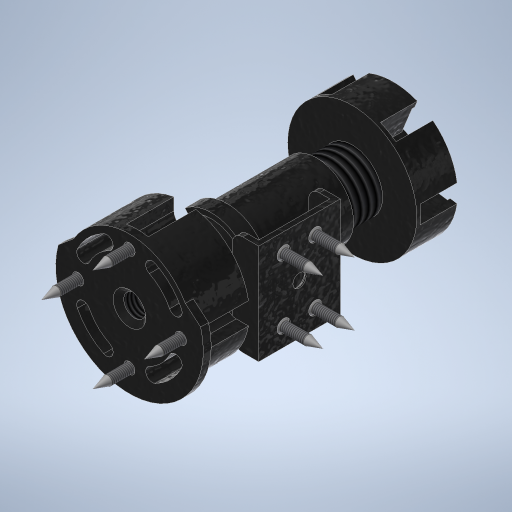
# Autodesk Inventor part: Adjustable leg  BT18 clip included
Saved by Autodesk Inventor 2024 (Build 280153000, 153)
## iProperties
Perskaiciuoti: 1
Category: Legs and supports
Created: 2006-11-23
Document SubType Name: Modeling
Designer: G.K.
Description: Adjustable leg
Authority: Design by UAB Čeli APS
Part Number: Adjustable leg  BT18 clip included
Mass: 31.9573 g
Surface Area: 217.096 cm^2
Volume: 31.9573 cm^3
Density: 1 g/cm^3
Material: Generic
Appearance: Fine Textured - Black
Pavadinimas: Koja
Šifras: Koja 001
Mase: 0.03195727
Author: G.K.
Title: Ajustable leg
Subject: Legs
Keywords: leg, adjustable, black
Comments: Ajustable leg, adjustable, black
Revision Number: 1
Autodesk Inventor part; units mm, degrees
ref_plane "YZ Plane" through (0, 0, 0) normal (1, 0, 0) x (0, 1, 0)
sketch "Sketch1" plane through (0, 0, 0) normal (1, 0, 0) x (0, 1, 0)
  line L0 (-14.2, 0) -> (85.2, 0) projected
  line L1 (0, 33.6) -> (0, -5.6) projected
  line L2 (71, 10.5) -> (71, 14)
  line L3 (71, 14) -> (21, 14)
  line L4 (21, 14) -> (21, 24.5)
  line L5 (21, 24.5) -> (3, 24.5)
  line L6 (3, 24.5) -> (3, 28)
  line L7 (3, 28) -> (0, 28)
  line L8 (0, 28) -> (0, 0)
  line L9 (71, 10.5) -> (53, 10.5)
  line L10 (53, 10.5) -> (53, 12)
  line L11 (53, 12) -> (3, 12)
  line L12 (3, 12) -> (3, 7)
  line L13 (3, 7) -> (9, 7)
  line L14 (9, 7) -> (9, 0)
  dimension "d139" = 24
  dimension "d0" = 71
  dimension "d1" = 68
  dimension "d2" = 18
  dimension "d3" = 56
  dimension "d4" = 49
  dimension "d5" = 3
  dimension "d6" = 21
  dimension "d7" = 28
  dimension "d8" = 21
  dimension "d9" = 24
  dimension "d11" = 62
  dimension "d12" = 14
  constraints: 26 end point, 6 parallel, 5 perpendicular, 4 point on line, 1 vertical
  measures "d0" distance between parallel lines of L2 L1
  measures "d1" distance between parallel lines of L12 L2
  measures "d2" distance of L2.start L9.end
  measures "d3" diameter of L7 L0
  measures "d4" diameter of L5 L0
  measures "d5" distance between parallel lines of L6 L8
  measures "d6" distance between parallel lines of L4 L8
  measures "d7" diameter of L3 L0
  measures "d8" diameter of L9 L0
  measures "d9" diameter of L11 L0
  measures "d11" distance between parallel lines of L14 L2
  measures "d12" diameter of L13 L0
revolve "Revolution1" add sketch "Sketch1" angle 360 about axis through (0, 0, 0) along (0, 1, 0)
sketch "Sketch2" plane through (0, 21, 0) normal (0, 1, 0) x (1, 0, 0)
  circle A0 centre (0, 0) radius 24.5 projected
  circle A1 centre (0, 0) radius 19.5 construction
  line L0 (0, 39.2) -> (0, -39.2) projected
  point P0 (0, 19.5)
  dimension "d14" = 39
  constraints: 1 coincident, 1 point on line, 1 vertical alignment, 2 other
hole "Hole1" at (0, 21, -19.5) direction (0, -1, 0) diameter 4.3 end through all
sketch "Sketch3" plane through (0, 21, 0) normal (0, 1, 0) x (1, 0, 0)
  circle A0 centre (0, 19.5) radius 2.15 projected
  circle A1 centre (0, 0) radius 24.5 projected
  arc A2 (-4.15, 19.5) -> (4.15, 19.5) centre (0, 19.5) ccw
  line L0 (-4.15, 19.5) -> (-4.15, 24.146)
  line L1 (4.15, 19.5) -> (4.15, 24.146)
  dimension "d22" = 8.3
  constraints: 4 end point, 4 point on circle, 2 tangent, 1 centre point, 1 coincident, 1 parallel, 1 vertical
  measures "d22" distance between parallel lines of L1 L0
extrude "Extrusion1" cut sketch "Sketch3" against normal blind 18 contours L1 A2 L0 A1 picked at (-3.4012, 21.3817)
hole "Hole2" at (0, 0, 0) direction (0, 1, 0) diameter 8.376 depth 20 tip angle 118 thread size "M10x1.5" class "6H" standard "ISO Metric profile"
thread "Thread1" size "M22x3" class "6H" standard "ISO Metric profile" full length
sketch "Sketch4" plane through (0, 0, 0) normal (0, -1, 0) x (1, 0, 0)
  circle A0 centre (0, 0) radius 28 projected
  arc A1 (7.1625, -20.8014) -> (20.8014, -7.1625) centre (0, 0) ccw
  arc A2 (5.5347, -16.0738) -> (16.0738, -5.5347) centre (0, 0) ccw
  arc A3 (4.15, -24.146) -> (24.146, -4.15) centre (0, 0) ccw projected
  line L0 (0, 39.2) -> (0, -39.2) projected
  line L1 (16.0738, -5.5347) -> (20.8014, -7.1625)
  line L2 (5.5347, -16.0738) -> (7.1625, -20.8014)
  line L3 (16.0738, -5.5347) -> (0, 0) construction
  line L4 (0, 0) -> (5.5347, -16.0738) construction
  dimension "d39" = 5
  dimension "d40" = 2.5
  dimension "d43" = 52
  dimension "d44" = 19
  constraints: 8 end point, 5 point on circle, 2 centre point, 2 coincident, 2 collinear, 1 point on line
  measures "d39" radial gap between concentric circles of A1 A2
  measures "d40" radial gap between concentric circles of A1 A3
  measures "d43" angle of L4 L3
  measures "d44" angle of L0 L4
extrude "Extrusion2" cut sketch "Sketch4" against normal blind 18 contours L2 A2 L1 A1
full round fillet "Fillet1" first side at (8.7138, 6, -20.2008) centre faces at (19.2255, 6, -6.6199) second side at (6.7334, 12, -15.6097)
full round fillet "Fillet2" first side at (8.4969, 6, -20.2929) centre faces at (6.0773, 6, -17.6497) second side at (14.7098, 6, -8.5219)
pattern_circular "Circular Pattern2" count 4 over 360 about axis through (0, 46, 0) along (0, -1, 0) of "Hole1", "Extrusion1", "Extrusion2", "Fillet1", "Fillet2"
chamfer "Chamfer1" distance 2 angle 45 1 edges at (0, 0, 4.188)
sketch "Sketch5" plane through (0, 3, 0) normal (0, 1, 0) x (1, 0, 0)
  arc A0 (24.146, 4.15) -> (4.15, 24.146) centre (0, 0) ccw projected
  line L0 (24.146, 4.15) -> (19.5, 4.15) projected
  arc A1 (-24.146, -4.15) -> (-4.15, -24.146) centre (0, 0) ccw projected
  line L1 (-24.146, -4.15) -> (-19.5, -4.15) projected
  line L2 (-19.5, 4.15) -> (-24.146, 4.15) projected
  circle A2 centre (0, 0) radius 28 projected
  line L3 (-27, -7.4162) -> (-21.1972, -12.2853)
  line L4 (0, 39.2) -> (0, -39.2) projected
  line L5 (27, -7.4162) -> (21.1972, -12.2853)
  arc A3 (-21.1972, -12.2853) -> (21.1972, -12.2853) centre (0, 0) ccw
  arc A4 (-27, -7.4162) -> (27, -7.4162) centre (0, 0) ccw
  dimension "d53" = 27
  dimension "d54" = 50
  constraints: 7 end point, 6 point on circle, 2 centre point, 2 coincident, 2 symmetric about line, 2 other
  measures "d53" distance from line of L4 L3.start
  measures "d54" angle of L3 L4
extrude "Extrusion3" cut sketch "Sketch5" against normal through all contours A1 A3 L4 A2 L3 | A3 L5 A2 L4 picked at (-24.3219, -10.92) picked at (24.3219, -10.92)
sketch "Sketch6" plane through (0, 0, 0) normal (0, 0, 1) x (1, 0, 0)
  line L0 (0, 22.894) -> (0, 122.294)
  line L1 (-28.3275, 84.5) -> (5.9725, 84.5)
  line L2 (-11.5, 29) -> (-11.5, 84.5)
  line L3 (-11.5, 84.5) -> (-24.5, 84.5)
  line L4 (-24.5, 84.5) -> (-24.5, 86)
  line L5 (-24.5, 86) -> (-11.5, 86)
  line L6 (-11.5, 86) -> (-11.5, 100)
  line L7 (-11.5, 100) -> (-9.25, 100)
  line L8 (-9.25, 100) -> (-9.25, 86)
  line L9 (-9.25, 86) -> (0, 86)
  line L10 (0, 84.5) -> (-9.5, 84.5)
  line L11 (-9.5, 84.5) -> (-9.5, 29)
  line L12 (-9.5, 29) -> (-11.5, 29)
  line L13 (0, 84.5) -> (0, 86)
  line L14 (14, 71) -> (-14, 71) projected
  point P0 (0, 0)
  dimension "d57" = 23
  dimension "d58" = 18.5
  dimension "d59" = 19
  dimension "d60" = 71
  dimension "d61" = 14
  dimension "d62" = 49
  dimension "d63" = 1.5
  dimension "d64" = 23
  dimension "d68" = 13.5
  constraints: 28 end point, 6 parallel, 5 collinear, 4 perpendicular, 3 point on line
  measures "d57" diameter of L2 L0
  measures "d58" diameter of L8 L0
  measures "d59" diameter of L11 L0
  measures "d60" distance between parallel lines of L12 L7
  measures "d61" distance between parallel lines of L7 L5
  measures "d62" diameter of L4 L0
  measures "d63" distance between parallel lines of L5 L1
  measures "d64" diameter of L6 L0
  measures "d68" distance between parallel lines of L3 L14
revolve "Revolution2" add sketch "Sketch6" angle 360 about axis through (0, 22.894, 0) along (0, 1, 0) separate body contours L1 L4 L5 L6 L7 L8 L9 L0 | L11 L14 L2 L1 | L11 L12 L2 L14
thread "Thread2" size "M24x3" class "6g" standard "ANSI Metric M Profile" full length
sketch "Sketch7" plane through (0, 86, 0) normal (0, 1, 0) x (1, 0, 0)
  circle A0 centre (0, 0) radius 11.5
  circle A1 centre (0, 0) radius 24.5
  arc A2 (7.2068, 21.8417) -> (-7.2068, 21.8417) centre (0, 0) ccw
  line L0 (-5.3569, 13.2587) -> (-9.1779, 22.716)
  line L1 (5.3369, 13.2093) -> (9.1779, 22.716)
  line L2 (-5.3569, 13.2587) -> (0, 0) construction
  line L3 (0, 0) -> (5.3369, 13.2093) construction
  line L4 (-5.3569, 13.2587) -> (-4.308, 10.6626)
  line L5 (5.3369, 13.2093) -> (4.308, 10.6626)
  line L6 (7.2068, 21.8417) -> (2.8804, 11.1334)
  line L7 (-7.2068, 21.8417) -> (-2.8804, 11.1334)
  dimension "d72" = 1.5
  dimension "d73" = 44
  dimension "d74" = 1.5
  dimension "d75" = 1.5
  constraints: 16 end point, 8 point on circle, 3 centre point, 2 collinear, 2 parallel, 2 point on line, 1 coincident
  measures "d72" radial gap between concentric circles of A2 A1
  measures "d73" angle of L3 L2
  measures "d74" distance between parallel lines of L5 L6
  measures "d75" distance between parallel lines of L7 L2
extrude "Extrusion4" add sketch "Sketch7" along normal up to surface (14 mm away) contours A0 L6 A2 L7 L4 L0 A1 L1 L5 bodies 2
pattern_circular "Circular Pattern3" count 6 over 360 about axis through (0, 85.25, 0) along (0, 1, 0) of "Extrusion4" bodies 2
sketch "Sketch8" plane through (0, 0, 0) normal (1, 0, 0) x (0, 1, 0)
  line L0 (99, 21.8417) -> (105.0942, 21.8417)
  line L1 (105.0942, 21.8417) -> (105.0942, 11.5)
  line L2 (105.0942, 11.5) -> (99, 11.5)
  line L3 (99, 11.5) -> (99, 21.8417)
  line L4 (86, 11.5) -> (100, 11.5) projected
  line L5 (100, 11.1334) -> (100, 21.8417) projected
  line L6 (86, 21.8417) -> (100, 21.8417) projected
  line L7 (-21.0188, 0) -> (126.113, 0) projected
  point P0 (0, 0)
  dimension "d81" = 1
  constraints: 8 end point, 2 collinear, 2 parallel, 1 horizontal, 1 perpendicular
  measures "d81" distance between parallel lines of L3 L5
revolve "Revolution3" cut sketch "Sketch8" angle 360 about axis through (0, -10, 0) along (0, 1, 0) bodies 2
revolve "Revolution4" [suppressed]
sketch "Sketch10" plane through (0, -24.4, 0) normal (0, -1, 0) x (1, 0, 0)
  circle A0 centre (0, 0) radius 8 projected
  line L0 (9.2376, -0.0209) -> (4.6007, -8.0104)
  line L1 (4.6007, -8.0104) -> (-4.6369, -7.9895)
  line L2 (-4.6369, -7.9895) -> (-9.2376, 0.0209)
  line L3 (-9.2376, 0.0209) -> (-4.6007, 8.0104)
  line L4 (-4.6007, 8.0104) -> (4.6369, 7.9895)
  line L5 (4.6369, 7.9895) -> (9.2376, -0.0209)
  constraints: 12 end point, 1 coincident, 1 tangent, 13 other
extrude "Extrusion5" [suppressed]
thread "Thread3" size "M10x1.5" class "6g" standard "ANSI Metric M Profile" full length
sketch "Sketch14" plane through (0, -18, 0) normal (0, 1, 0) x (1, 0, 0)
  circle A0 centre (0, 0) radius 5 projected
  circle A1 centre (0, 0) radius 7.25 projected
  circle A2 centre (0, 0) radius 5
  dimension "d102" = 10
  constraints: 1 centre point, 1 coincident
  measures "d102" diameter of A2
extrude "Extrusion6" [suppressed]
sketch "Sketch15" plane through (0, 0, 0) normal (1, 0, 0) x (0, 1, 0)
  line L0 (3, -23.7) -> (3, -18.8) construction
  line L1 (6.6298, -19.5) -> (-17.1702, -19.5)
  line L2 (3, -19.5) -> (3, -23)
  line L3 (3, -23) -> (2.5, -23)
  line L4 (2.5, -23) -> (0.75, -21.25)
  line L5 (0.75, -21.25) -> (-8.276, -21.25)
  line L6 (-8.276, -21.25) -> (-14, -19.5)
  line L7 (0, -21.65) -> (0, -17.35) projected
  line L8 (0, -19.5) -> (3.4682, -19.5) construction
  line L9 (3, -24.146) -> (3, -19.5) projected
  point P0 (0, 0)
  dimension "d105" = 3.5
  dimension "d106" = 7
  dimension "d107" = 0.5
  dimension "d108" = 45
  dimension "d109" = 17
  dimension "d110" = 17
  dimension "d111" = 9.026
  constraints: 16 end point, 3 collinear, 3 perpendicular, 2 point on line, 1 midpoint, 1 parallel
  measures "d105" diameter of L5 L1
  measures "d106" diameter of L3 L1
  measures "d107" distance from line of L3.end L2
  measures "d108" angle of L4 L2
  measures "d109" distance from line of L6.end L2
  measures "d110" angle of L6 L1
  measures "d111" distance of L4.end L5.end
revolve "Revolution8" add sketch "Sketch15" angle 360 about axis through (0, 6.6298, -19.5) along (0, -1, 0) separate body
sketch "Sketch16" plane through (0, 0, 0) normal (1, 0, 0) x (0, 1, 0)
  line L0 (0.84, -19.5) -> (3.36, -19.5)
  line L1 (1.2, -19.5) -> (1.2, -18.5104)
  line L2 (1.2, -18.5104) -> (3, -17)
  line L3 (3, -17) -> (3, -19.5)
  line L4 (3, -21.65) -> (3, -17.35) projected
  point P0 (0, 0)
  point P1 (3, -19.5)
  dimension "d113" = 40
  dimension "d114" = 1.8
  dimension "d115" = 2.5
  constraints: 8 end point, 2 perpendicular, 2 point on line, 1 midpoint
  measures "d113" angle of L2 L0
  measures "d114" distance between parallel lines of L1 L3
  measures "d115" distance from line of L0 L2.end
extrude "Extrusion7" cut sketch "Sketch16" along normal mid plane 1 bodies 3
pattern_circular "Circular Pattern4" count 4 over 360 about axis through (0, -3.763, -19.5) along (0, -1, 0) of "Extrusion7" bodies 3
thread "Thread4" size "M4x0.7" class "6g" standard "ANSI Metric M Profile" full length
ref_plane "Work Plane2" through (0, 31, 0) normal (0, -1, 0) x (1, 0, 0)
sketch "Sketch18" plane through (0, 31, 0) normal (0, -1, 0) x (1, 0, 0)
  arc A0 (-8.6603, -11) -> (-8.6603, 11) centre (0, 0) ccw
  arc A1 (-9.8974, -12.5714) -> (-9.8974, 12.5714) centre (0, 0) ccw
  line L0 (18, -10) -> (18, 10)
  line L1 (14, -6.4724) -> (14, 14.1834) construction
  line L2 (21, 10) -> (21, -10) construction
  line L3 (18, -7.5) -> (14.1333, -7.5)
  line L4 (14.1333, 7.5) -> (18, 7.5)
  line L5 (27.1795, 0) -> (0, 34.0769) construction
  line L6 (-8.6603, -11) -> (-9.8974, -12.5714)
  line L7 (-8.6603, 11) -> (-9.8974, 12.5714)
  point P0 (0, 0)
  point P1 (18, 0)
  point P2 (18, 0)
  point P3 (27.1795, 0)
  point P4 (0, 34.0769)
  dimension "d129" = 2
  dimension "d130" = 28
  dimension "d131" = 7
  dimension "d132" = 15
  dimension "d133" = 22
  constraints: 14 end point, 6 point on circle, 3 point on line, 2 centre point, 2 perpendicular, 1 coincident, 1 midpoint, 1 parallel, 1 tangent, 3 other
  measures "d129" radial gap between concentric circles of A1 A0
  measures "d130" diameter of A0
  measures "d131" distance between parallel lines of L1 L2
  measures "d132" distance between parallel lines of L4 L3
  measures "d133" distance of L7.start L6.start
extrude "Extrusion8" add sketch "Sketch18" against normal blind 6 separate body
sketch "Sketch19" plane through (0, 31, 0) normal (0, -1, 0) x (1, 0, 0)
  line L0 (18, -7.5) -> (18, 7.5) projected
  arc A0 (14.1333, 7.5) -> (-9.8974, 12.5714) centre (0, 0) ccw projected
  line L1 (21, 10) -> (18, 10)
  line L2 (18, 10) -> (18, -10)
  line L3 (18, -10) -> (21, -10)
  line L4 (21, -10) -> (21, 10)
  point P0 (21, 0)
  dimension "d136" = 20
  dimension "d137" = 3
  constraints: 8 end point, 2 parallel, 1 collinear, 1 horizontal, 1 horizontal alignment, 1 midpoint, 1 perpendicular
  measures "d136" distance of L3.end L1.start
  measures "d137" distance of L1.start L1.end
extrude "Extrusion9" add sketch "Sketch19" along normal blind 3 and the other way blind 24 bodies 4
sketch "Sketch20" plane through (0, 28, 0) normal (0, -1, 0) x (1, 0, 0)
  line L0 (18, 10) -> (18, -10) projected
  line L1 (23, 19) -> (17, 19)
  line L2 (13, 15) -> (13, -15)
  line L3 (17, -19) -> (23, -19)
  line L4 (23, -19) -> (23, 19)
  arc A0 (17, 19) -> (13, 15) centre (17, 15) ccw
  arc A1 (13, -15) -> (17, -19) centre (17, -15) ccw
  point P0 (0, 0)
  point P1 (13, -19)
  point P2 (13, 19)
  point P3 (23, 0)
  dimension "d142" = 10
  dimension "d143" = 38
  dimension "d144" = 5
  dimension "d145" = 4
  constraints: 8 end point, 4 point on circle, 4 point on line, 4 tangent, 2 centre point, 2 parallel, 1 equal radius, 1 horizontal, 1 horizontal alignment, 1 midpoint, 1 perpendicular
  measures "d142" distance of L3.end point (13, -19)
  measures "d143" distance of point (13, -19) point (13, 19)
  measures "d144" distance between parallel lines of L4 L0
  measures "d145" radius of A0
extrude "Extrusion10" add sketch "Sketch20" along normal blind 2 and the other way blind 29 separate body
sketch "Sketch21" plane through (23, 26, -19) normal (0, 0, -1) x (-1, 0, 0)
  line L0 (0, 31) -> (0, 0) projected
  line L1 (6, 0) -> (0, 0) projected
  line L2 (0, 31) -> (6, 31) projected
  line L3 (2, 29) -> (13.1026, 29)
  line L4 (13.1026, 29) -> (13.1026, 2)
  line L5 (13.1026, 2) -> (2, 2)
  line L6 (2, 2) -> (2, 29)
  point P0 (23, -26)
  dimension "d150" = 2
  dimension "d151" = 2
  dimension "d152" = 2
  constraints: 8 end point, 2 parallel, 1 horizontal, 1 perpendicular
  measures "d150" distance between parallel lines of L5 L1
  measures "d151" distance between parallel lines of L2 L3
  measures "d152" distance between parallel lines of L0 L6
extrude "Extrusion11" cut sketch "Sketch21" against normal through all bodies 5
sketch "Sketch22" plane through (21, 28, -19) normal (-1, 0, 0) x (0, 0, 1)
  line L0 (38, 27) -> (38, 0) projected
  line L1 (7, 19.5) -> (31, 19.5)
  line L2 (31, 19.5) -> (31, 7.5)
  line L3 (31, 7.5) -> (7, 7.5)
  line L4 (7, 7.5) -> (7, 19.5)
  line L5 (7, 19.5) -> (31, 7.5) construction
  line L6 (31, 19.5) -> (7, 7.5) construction
  line L7 (34, 0) -> (4, 0) projected
  point P0 (19, -28)
  point P1 (19, 13.5)
  point P2 (19, 13.5)
  point P3 (19, 0)
  point P4 (19, 13.5)
  point P5 (38, 13.5)
  dimension "d155" = 24
  dimension "d156" = 12
  constraints: 12 end point, 6 midpoint, 2 parallel, 1 horizontal, 1 horizontal alignment, 1 perpendicular, 1 vertical alignment
  measures "d155" distance of L2.end L3.end
  measures "d156" distance of L1.end L2.end
hole "Hole3" at (21, 35.5, -12) at (21, 41.5, 0) at (21, 47.5, -12) at (21, 47.5, 12) at (21, 35.5, 12) direction (1, 0, 0) diameter 5 end through all countersink diameter 8 countersink angle 90 bodies 5
ref_plane "Work Plane3" through (71.05, 47.5, -12) normal (0, 0, -1) x (-1, 0, 0)
sketch "Sketch23" plane through (71.05, 47.5, -12) normal (0, 0, -1) x (-1, 0, 0)
  line L0 (50.05, -4.2) -> (50.05, 0.7) construction
  line L1 (53.45, 0) -> (29.65, 0)
  line L2 (50.05, 0) -> (50.05, -3.5)
  line L3 (50.05, -3.5) -> (49.55, -3.5)
  line L4 (49.55, -3.5) -> (47.8, -1.75)
  line L5 (47.8, -1.75) -> (38.774, -1.75)
  line L6 (38.774, -1.75) -> (33.05, 0)
  line L7 (50.05, 4) -> (50.05, -4) projected
  point P0 (71.05, -47.5)
  point P1 (50.05, 0)
  dimension "d165" = 3.5
  dimension "d166" = 7
  dimension "d167" = 0.5
  dimension "d168" = 45
  dimension "d169" = 17
  dimension "d170" = 17
  dimension "d171" = 9.026
  constraints: 14 end point, 2 perpendicular, 2 point on line, 1 collinear, 1 midpoint, 1 parallel
  measures "d165" diameter of L5 L1
  measures "d166" diameter of L3 L1
  measures "d167" distance from line of L3.end L2
  measures "d168" angle of L4 L2
  measures "d169" distance from line of L6.end L2
  measures "d170" angle of L6 L1
  measures "d171" distance of L4.end L5.end
revolve "Revolution9" add sketch "Sketch23" angle 360 about axis through (17.6, 47.5, -12) along (1, 0, 0) separate body
sketch "Sketch24" plane through (71.05, 47.5, -12) normal (0, 0, -1) x (-1, 0, 0)
  line L0 (47.89, 0) -> (50.41, 0)
  line L1 (48.25, 0) -> (48.25, 0.9896)
  line L2 (48.25, 0.9896) -> (50.05, 2.5)
  line L3 (50.05, 2.5) -> (50.05, 0)
  line L4 (50.05, 3.5) -> (50.05, -3.5)
  line L5 (50.05, 3.5) -> (50.05, -3.5) projected
  point P0 (71.05, -47.5)
  point P1 (50.05, 0)
  dimension "d173" = 40
  dimension "d174" = 1.8
  dimension "d175" = 2.5
  constraints: 10 end point, 2 perpendicular, 2 point on line, 1 collinear, 1 midpoint
  measures "d173" angle of L2 L0
  measures "d174" distance between parallel lines of L1 L3
  measures "d175" distance from line of L0 L2.end
extrude "Extrusion12" cut sketch "Sketch24" along normal mid plane 1 bodies 6
pattern_circular "Circular Pattern6" count 4 over 360 about axis through (27.763, 47.5, -12) along (1, 0, 0) of "Extrusion12" bodies 6
thread "Thread5" size "M4x0.7" class "6g" standard "ANSI Metric M Profile" full length
pattern_linear "Rectangular Pattern1" count 2 spacing 12 along (0, -1, 0) count 2 spacing 24 along (0, 0, 1) bodies 6
ref_plane "Work Plane4" through (-2.3003, -24.4, 4.0052) normal (0.867154, 0, 0.4980402) x (0.4980402, 0, -0.867154)
revolve "Revolution10" [suppressed]
pattern_circular "Circular Pattern7" count 4 over 360 about axis through (0, -10, 0) along (0, 1, 0) bodies 3
sketch "Sketch9" plane through (0, 0, 0) normal (1, 0, 0) x (0, 1, 0)
  line L0 (-24.4, 0) -> (12, 0)
  line L1 (12, 0) -> (12, 4)
  line L2 (11, 5) -> (-18, 5)
  line L3 (-18, 5) -> (-18, 7.25)
  line L4 (-18, 7.25) -> (-18.6, 7.25)
  line L5 (-18.6, 7.25) -> (-18.6, 8)
  line L6 (-18.6, 8) -> (-24.4, 8)
  line L7 (-24.4, 8) -> (-24.4, 0)
  line L8 (0, 15.2316) -> (0, 7.5497) projected
  line L9 (11, 5) -> (12, 4)
  point P0 (0, 0)
  point P1 (12, 5)
  dimension "d83" = 30
  dimension "d84" = 0.6
  dimension "d85" = 10
  dimension "d86" = 18
  dimension "d87" = 14.5
  dimension "d88" = 5.8
  dimension "d89" = 16
  dimension "d90" = 1
  dimension "d91" = 1
  constraints: 20 end point, 4 parallel, 3 perpendicular, 3 point on line, 1 horizontal
  measures "d83" distance between parallel lines of L3 L1
  measures "d84" distance from line of L4.end L3
  measures "d85" diameter of L2 L0
  measures "d86" distance between parallel lines of L3 L8
  measures "d87" diameter of L4.end L0
  measures "d88" distance between parallel lines of L7 L5
  measures "d89" diameter of L6 L0
  measures "d90" distance of L2.start point (12, 5)
  measures "d91" distance of L1.end point (12, 5)
sketch "Sketch25" plane through (-2.3003, -24.4, 4.0052) normal (0.867154, 0, 0.4980402) x (0.4980402, 0, -0.867154)
  line L0 (-5.1097, -0.7289) -> (-1.8613, -0.7289)
  line L1 (-1.8613, -0.7289) -> (-5.1097, 1.1642)
  line L2 (-5.1097, 1.1642) -> (-5.1097, -0.7289)
  line L3 (0, 0) -> (-4.6188, 0) projected
  line L4 (4.6188, -25.7547) -> (4.6188, 149.4258) projected
  point P0 (4.6188, 24.4)
  dimension "d192" = 0.7289
  dimension "d193" = 0.4909
  constraints: 6 end point, 1 horizontal, 1 vertical
  measures "d192" distance between parallel lines of L0 L3
  measures "d193" distance from line of L3.end L2
equation "\"d86\" = Bottom_board_thickness"
equation "\"d91\" = d90"
equation "\"Bottom_board_thickness\" = 18"
